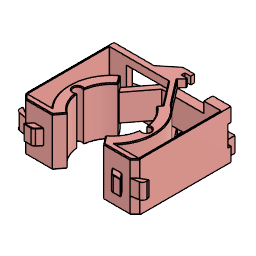
omega clamp - AS5311 (Autodesk Fusion 360 design; units mm, degrees)
Autodesk Fusion 360 part; units mm, degrees
sketch "Sketch1" plane through (0, 0, 0) normal (0, 0, 1) x (1, 0, 0)
  arc A0 (-9.9403, 13.1697) -> (-16.4122, 1.6998) centre (0, 0) ccw
  arc A1 (-16.4122, 1.6998) -> (-16.4122, -1.6998) centre (-17.8088, 0) ccw
  arc A2 (-16.4122, -1.6998) -> (-9.9403, -13.1697) centre (0, 0) ccw
  line L0 (0, 0) -> (-44, 0) construction
  arc A3 (-13.259, 17.5667) -> (-13.259, -17.5667) centre (0, 0) ccw
  line L1 (-9.9403, -13.1697) -> (-13.259, -17.5667)
  line L2 (-9.9403, 13.1697) -> (-13.259, 17.5667)
  line L3 (0, 0) -> (-9.9403, -13.1697) construction
  line L4 (0, 0) -> (-9.9403, 13.1697) construction
  point P0 (-20.0088, 0)
  point P1 (-16.0088, 0)
  point P2 (-22.0088, 0)
  dimension "d12" = 2.2
  dimension "d14" = 4
  dimension "d15" = 2
  dimension "d80" = 33
  dimension "d82" = 3.3997
  dimension "d83" = 105.91
  constraint coincident A0.centre A2.centre
  constraint horizontal L0
  constraint coincident A1.centre L0
  constraint midpoint A1 P0
  constraint coincident L0 P1
  constraint coincident L0 P2
  constraint coincident A3 P2
  constraint midpoint A3 P2
  constraint coincident A0.centre L1
  constraint parallel L2 L4
  constraint equal A0 A2
  measures "d12" radius of A1
  measures "d14" distance of P0 P1
  measures "d15" distance of P0 P2
  measures "d80" diameter of A0
  measures "d82" distance of A0.end A1.end
  measures "d83" angle of L3 L4
extrude "Extrude1" add sketch "Sketch1" along normal blind 25 makes body 1
mirror "Mirror1" about plane through (0, 0, 0) normal (1, 0, 0) of bodies 1 makes body 2
sketch "Sketch2" plane through (0, 0, 0) normal (0, 0, 1) x (1, 0, 0)
  arc A0 (-13.259, 17.5667) -> (-13.259, -17.5667) centre (0, 0) ccw
  arc A1 (-16.4122, -1.6998) -> (-9.9403, -13.1697) centre (0, 0) ccw
  arc A2 (-16.4122, 1.6998) -> (-16.4122, -1.6998) centre (-17.8088, 0) ccw
  arc A3 (-9.9403, 13.1697) -> (-16.4122, 1.6998) centre (0, 0) ccw
  arc A4 (16.4122, 1.6998) -> (9.9403, 13.1697) centre (0, 0) ccw
  arc A5 (16.4122, -1.6998) -> (16.4122, 1.6998) centre (17.8088, 0) ccw
  arc A6 (9.9403, -13.1697) -> (16.4122, -1.6998) centre (0, 0) ccw
  arc A7 (13.259, -17.5667) -> (13.259, 17.5667) centre (0, 0) ccw
  line L0 (-13.259, -17.5667) -> (-29.4985, -17.5667)
  line L1 (-29.4985, -17.5667) -> (-29.4985, -14.5667)
  line L2 (-29.4985, -14.5667) -> (-16.4985, -14.5667)
  line L3 (-29.4985, -14.5667) -> (-29.4985, 27.5667)
  line L4 (-28.8485, 27.5667) -> (-28.8485, -14.5667)
  line L5 (-29.4985, 27.5667) -> (1.7818, 27.5667)
  line L6 (-29.4985, 27.5667) -> (-29.4985, 30.5667)
  line L7 (-29.4985, 30.5667) -> (3.259, 30.5667)
  line L8 (3.259, 30.5667) -> (13.259, 17.5667)
  line L9 (1.7818, 27.5667) -> (11.3845, 15.0832)
  line L10 (-13.259, -17.5667) -> (-6.9615, -17.5667)
  line L11 (-26.9985, -17.5667) -> (-29.4985, -15.0667)
  line L12 (-6.9615, -17.5667) -> (36, -17.5667)
  line L13 (-9.9403, 13.1697) -> (-13.259, 17.5667)
  line L14 (-13.259, -17.5667) -> (-9.9403, -13.1697)
  line L15 (9.9403, -13.1697) -> (13.259, -17.5667)
  line L16 (13.259, 17.5667) -> (9.9403, 13.1697)
  dimension "d40" = 3
  dimension "d41" = 0.65
  dimension "d42" = 3
  dimension "d43" = 3
  dimension "d45" = 10
  dimension "d46" = 10
  dimension "d47" = 42.1333
  dimension "d48" = 13
  dimension "d49" = 45
  dimension "d50" = 0.5
  constraint horizontal L0
  constraint perpendicular L0 L1
  constraint coincident A0 L2.end
  constraint perpendicular L1 L2
  constraint perpendicular L2 L3
  constraint coincident L2 L4.end
  constraint perpendicular L2 L4
  constraint perpendicular L4 L5
  constraint coincident L4.start L5
  constraint perpendicular L5 L6
  constraint perpendicular L6 L7
  constraint coincident A7.end L8.end
  constraint parallel L8 L9
  constraint horizontal L10
  constraint coincident L0 L11.start
  constraint coincident L1 L11.end
  constraint parallel L10 L12
  constraint coincident L9.end L16
  constraint coincident A0.end L0.start
  measures "d40" distance of L0.end L1.end
  measures "d41" distance of L3 L4
  measures "d42" distance of L8 L9
  measures "d43" distance of L5 L7
  measures "d45" horizontal distance of L7.end A7.end
  measures "d46" vertical distance of A0.start L5.end
  measures "d47" distance of L1.end L3.end
  measures "d48" distance of L1.end L2.end
  measures "d49" angle of L0 L11
  measures "d50" distance of L1.end L11.end
extrude "Extrude2" add sketch "Sketch2" along normal up to surface (25 mm away) separate body contours A0 L0 L1 L2 L11 | L2 L3 L4 L5 | L5 L6 L7 L8 L9 L16 makes body 3
ref_plane "WorkPlane3" through (-8.1198, 6.5, 12.5) normal (0, 0, 1) x (1, 0, 0)
sketch "Sketch4" plane through (-6.4898, 5.5, 12.5) normal (0, 0, 1) x (1, 0, 0)
  line L0 (19.7488, 12.0667) -> (9.7488, 25.0667)
  line L1 (9.7488, 25.0667) -> (-23.0087, 25.0667)
  line L2 (-23.0087, 25.0667) -> (-23.0087, -20.5667)
  line L3 (-23.0087, -20.5667) -> (-20.5087, -23.0667)
  line L4 (-20.5087, -23.0667) -> (-6.7692, -23.0667)
  arc A0 (-10.0087, -20.0667) -> (-6.7692, -23.0667) centre (6.4898, -5.5) ccw
  line L5 (-20.5087, -23.0667) -> (-24.597, -22.3458)
  line L6 (-26.2193, -20.0289) -> (-26.0087, -18.8346)
  line L7 (-26.0087, -18.8346) -> (-23.0087, -20.5667)
  arc A1 (-26.2193, -20.0289) -> (-24.597, -22.3458) centre (-24.2497, -20.3762) ccw
  line L8 (17.8743, 9.5832) -> (19.7488, 12.0667)
  line L9 (-10.0087, -20.0667) -> (-22.3587, -20.0667)
  line L10 (-22.3587, -20.0667) -> (-22.3587, 22.0667)
  line L11 (-22.3587, 22.0667) -> (8.2716, 22.0667)
  line L12 (8.2716, 22.0667) -> (17.8743, 9.5832)
  line L13 (-16.2943, -23.0667) -> (-18.8116, -26.0667)
  line L14 (-18.8116, -26.0667) -> (-14.7443, -26.0667)
  arc A2 (-14.7443, -26.0667) -> (-13.2122, -25.3523) centre (-14.7443, -24.0667) ccw
  line L15 (-13.2122, -25.3523) -> (-11.2943, -23.0667)
  arc A3 (-18.5359, -25.7381) -> (-18.3827, -26.0667) centre (-18.3827, -25.8667) ccw
  dimension "d69" = 2
  dimension "d70" = 3
  dimension "d72" = 60
  dimension "d73" = 10
  dimension "d119" = 50
  dimension "d120" = 3
  dimension "d123" = 2
  dimension "d124" = 5
  dimension "d125" = 0.2
  constraint coincident L3.end L4.start
  constraint perpendicular L5 L6
  constraint coincident L2.end L3.start
  constraint tangent L5 A1
  constraint tangent L6 A1
  constraint coincident L4 L13.start
  constraint horizontal L14
  constraint tangent L14 A2
  constraint coincident L4 L15.end
  constraint parallel L13 L15
  constraint tangent A2 L15
  constraint tangent L13 A3
  constraint coincident L13 A3.start
  constraint coincident L14 A3.end
  constraint tangent L14 A3
  measures "d69" radius of A1
  measures "d70" horizontal distance of L6.end L2.end
  measures "d72" angle of L2 L7
  measures "d73" angle of L4 L5
  measures "d119" angle of L4 L13
  measures "d120" distance of L4 L13.end
  measures "d123" radius of A2
  measures "d124" distance of L13.start L15.end
  measures "d125" radius of A3
extrude "Extrude7" add sketch "Sketch4" along normal mid plane 8 contours L3 L5 L6 L7 A1 | L4 L13 L14 A2 L15 A3 bodies 3
mirror "Mirror2" about plane through (0, 0, 0) normal (1, 0, 0) of bodies 3 makes body 4
ref_plane "WorkPlane5" through (-13.1198, 30.5667, 12.5) normal (0, 1, 0) x (-1, 0, 0)
sketch "Sketch3" plane through (-13.1198, 30.5667, 12.5) normal (0, 1, 0) x (-1, 0, 0)
  line L0 (16.3787, -8.5) -> (-42.6183, -8.5)
  line L1 (16.3787, -6.9) -> (-42.6183, -6.9)
  line L2 (-42.6183, 6.9) -> (16.3787, 6.9)
  line L3 (16.3787, 8.5) -> (-43, 8.5)
  line L4 (-13.1198, -8.5) -> (-13.1198, -6.9) construction
  line L5 (-13.1198, -8.5) -> (-13.1198, -12.5) construction
  line L6 (6.8802, 12.5) -> (6.8802, -12.5)
  line L7 (-33.1198, -12.5) -> (-33.1198, 12.5)
  line L8 (-13.1198, -6.9) -> (-13.1198, 6.9) construction
  line L9 (-13.1198, 6.9) -> (-13.1198, 8.5) construction
  line L10 (-13.1198, 12.5) -> (-13.1198, 8.5) construction
  line L11 (-33.1198, -12.5) -> (6.8802, 12.5) construction
  line L12 (-42.6183, -12.5) -> (-42.6183, 12.5)
  line L13 (16.3787, -12.5) -> (16.3787, 12.5)
  line L14 (16.3787, -12.5) -> (-42.6183, -12.5)
  line L15 (-42.6183, 12.5) -> (16.3787, 12.5)
  point P0 (-13.1198, 0)
  dimension "d58" = 1.6
  dimension "d129" = 4
  dimension "d130" = 40
  constraint horizontal L2
  constraint vertical L4
  constraint vertical L5
  constraint coincident L2 L8.end
  constraint coincident L3 L9.end
  constraint vertical L6
  constraint vertical L7
  constraint coincident L0 L4.start
  constraint coincident L1 L4.end
  constraint equal L5 L10
  constraint equal L4 L9
  constraint vertical L8
  constraint vertical L9
  constraint vertical L10
  constraint midpoint L11 P0
  constraint coincident L8 P0
  constraint coincident L13.start L14.start
  constraint coincident L12.start L14.end
  constraint coincident L12.end L15.start
  constraint coincident L13.end L15.end
  constraint midpoint L5.end L14
  constraint horizontal L1
  constraint coincident L1.end L12
  constraint coincident L0.end L12
  constraint coincident L1.start L13
  constraint coincident L0.start L13
  constraint coincident L2.start L12
  constraint perpendicular L3 L12
  constraint midpoint L10.start L15
  constraint coincident L6.end L14
  constraint coincident L2.end L13
  constraint coincident L3.start L13
  constraint coincident L7.end L15
  constraint coincident L7.start L14
  constraint coincident L6.start L15
  measures "d58" distance of L0 L1
  measures "d129" distance of L4.start L5.end
  measures "d130" distance of L6 L7
extrude "Extrude5" cut sketch "Sketch3" against normal blind 20 contours L0 L6 L13 L14 | L0 L1 L6 L13 | L0 L6 L7 L14 | L0 L1 L6 L7 | L1 L2 L6 L13 | L2 L3 L6 L13 | L2 L3 L6 L7 | L3 L6 L13 L15 | L3 L6 L7 L15 bodies 4
extrude "Extrude6" cut sketch "Sketch3" against normal blind 25 contours L0 L1 L6 L7 | L1 L2 L6 L7 | L2 L3 L6 L7 bodies 3
combine "Combine1" operation add target body 1 tool bodies 2 3 4
sketch "Sketch5" plane through (0, 30.5667, 0) normal (0, 1, 0) x (-1, 0, 0)
  line L0 (-29.4985, 25) -> (-29.4985, 0)
  line L1 (-20, 0) -> (-20, 5.6)
  line L2 (-20, 5.6) -> (3.259, 5.6)
  line L3 (3.259, 5.6) -> (3.259, 19.4)
  line L4 (3.259, 19.4) -> (-20, 19.4)
  line L5 (3.259, 7.2) -> (-29.4985, 7.2)
  line L6 (3.259, 17.8) -> (-29.4985, 17.8)
  line L7 (3.259, 17.8) -> (-29.4985, 7.2) construction
  line L8 (-13.1198, 12.5) -> (3.259, 12.5) construction
  line L9 (-20, 25) -> (-29.4985, 25)
  line L10 (-29.4985, 0) -> (-20, 0)
  line L11 (-20, 19.4) -> (-20, 25)
  dimension "d84" = 10.6
  constraint coincident L3 L5.start
  constraint coincident L0 L5.end
  constraint perpendicular L0 L5
  constraint coincident L3 L6.start
  constraint coincident L0 L6.end
  constraint perpendicular L0 L6
  constraint midpoint L7 L8.start
  constraint midpoint L3 L8.end
  constraint horizontal L8
  measures "d84" distance of L5 L6
extrude "Extrude8" add sketch "Sketch5" along normal blind 1.6 contours L0 L3 L4 L6 L9 L11 | L0 L1 L2 L3 L5 L10 bodies 1
sketch "Sketch6" plane through (0, 0, 0) normal (0, 0, 1) x (1, 0, 0)
  line L0 (2.4985, 33.4667) -> (24.4985, 33.4667)
  line L1 (24.4985, 33.4667) -> (24.4985, 35.2667)
  line L2 (24.4985, 35.2667) -> (2.4985, 35.2667)
  line L3 (2.4985, 35.2667) -> (2.4985, 33.4667)
  line L4 (-3.259, 32.1667) -> (29.4985, 32.1667)
  line L5 (26.4985, 32.8667) -> (-29.4985, 32.8667)
  line L6 (-29.4985, 32.8667) -> (-29.4985, 37.2667)
  line L7 (-29.4985, 37.2667) -> (26.4985, 37.2667)
  line L8 (26.4985, 37.2667) -> (26.4985, 32.8667)
  arc A0 (-9.9403, 13.1697) -> (-16.4122, 1.6998) centre (0, 0) ccw
  arc A1 (-16.4122, 1.6998) -> (-16.4122, -1.6998) centre (-17.8088, 0) ccw
  arc A2 (-16.4122, -1.6998) -> (-9.9403, -13.1697) centre (0, 0) ccw
  line L9 (-9.9403, -13.1697) -> (-13.259, -17.5667)
  line L10 (-13.259, -17.5667) -> (-26.9985, -17.5667)
  line L11 (-26.9985, -17.5667) -> (-29.4985, -15.0667)
  line L12 (-29.4985, -15.0667) -> (-29.4985, 30.5667)
  line L13 (-29.4985, 30.5667) -> (3.259, 30.5667)
  line L14 (3.259, 30.5667) -> (13.259, 17.5667)
  arc A3 (16.4985, -14.5667) -> (13.259, 17.5667) centre (0, 0) ccw
  line L15 (16.4985, -14.5667) -> (28.8485, -14.5667)
  line L16 (28.8485, -14.5667) -> (28.8485, 27.5667)
  line L17 (28.8485, 27.5667) -> (20, 27.5667)
  line L18 (20, 27.5667) -> (20, 32.1667)
  line L19 (20, 32.1667) -> (29.4985, 32.1667)
  line L20 (29.4985, 32.1667) -> (29.4985, -15.0667)
  line L21 (29.4985, -15.0667) -> (26.9985, -17.5667)
  line L22 (26.9985, -17.5667) -> (13.259, -17.5667)
  line L23 (13.259, -17.5667) -> (9.9403, -13.1697)
  arc A4 (9.9403, -13.1697) -> (16.4122, -1.6998) centre (0, 0) ccw
  arc A5 (16.4122, -1.6998) -> (16.4122, 1.6998) centre (17.8088, 0) ccw
  arc A6 (16.4122, 1.6998) -> (9.9403, 13.1697) centre (0, 0) ccw
  line L24 (9.9403, 13.1697) -> (11.3845, 15.0832)
  line L25 (11.3845, 15.0832) -> (1.7818, 27.5667)
  line L26 (1.7818, 27.5667) -> (-28.8485, 27.5667)
  line L27 (-28.8485, 27.5667) -> (-28.8485, -14.5667)
  line L28 (-28.8485, -14.5667) -> (-16.4985, -14.5667)
  arc A7 (-13.259, 17.5667) -> (-16.4985, -14.5667) centre (0, 0) ccw
  line L29 (-13.259, 17.5667) -> (-9.9403, 13.1697)
  line L30 (-29.4985, 30.5667) -> (-29.4985, 32.8667)
  line L31 (3.259, 30.5667) -> (3.259, 32.8667)
  line L32 (-20, 30.5667) -> (-20, 27.5667)
  line L33 (-20, 30.5667) -> (-20, 32.8667)
  line L34 (-29.4985, 32.8667) -> (-9.4985, 37.2667)
  line L35 (18.4985, 35.2667) -> (18.4985, 33.4667)
  line L36 (8.4985, 33.4667) -> (8.4985, 35.2667)
  line L37 (8.4985, 33.4667) -> (18.4985, 35.2667) construction
  line L38 (13.4985, 34.3667) -> (13.4985, 35.2667) construction
  line L39 (5.4985, 32.8667) -> (5.4985, 33.4667)
  line L40 (5.4985, 35.2667) -> (5.4985, 37.2667)
  line L41 (-0.5015, 37.2667) -> (-8.741, 30.5667)
  line L42 (5.4985, 32.8667) -> (3.259, 30.5667)
  point P0 (3.259, 30.5667)
  dimension "d87" = 22
  dimension "d88" = 1.8
  dimension "d89" = 3.1
  dimension "d90" = 5
  dimension "d91" = 0.6
  dimension "d92" = 2
  dimension "d93" = 2
  dimension "d96" = 20
  dimension "d101" = 10
  dimension "d104" = 3
  dimension "d106" = 12
  dimension "d107" = 3
  constraint horizontal L0
  constraint vertical L1
  constraint horizontal L2
  constraint vertical L3
  constraint horizontal L5
  constraint vertical L6
  constraint horizontal L7
  constraint vertical L8
  constraint coincident L12.end L13.start
  constraint vertical L30
  constraint coincident P0 L13.end
  constraint coincident L5 L31.end
  constraint perpendicular L5 L31
  constraint coincident L5 L33.end
  constraint perpendicular L5 L33
  constraint coincident L32.start L33.start
  constraint coincident L7 L34.end
  constraint coincident L2 L35.start
  constraint coincident L0 L35.end
  constraint perpendicular L0 L35
  constraint coincident L0 L36.start
  constraint coincident L2 L36.end
  constraint perpendicular L2 L36
  constraint midpoint L37 L38.start
  constraint midpoint L2 L38.end
  constraint vertical L38
  constraint coincident L5 L39.start
  constraint coincident L0 L39.end
  constraint perpendicular L0 L39
  constraint coincident L2 L40.start
  constraint coincident L7 L40.end
  constraint perpendicular L7 L40
  constraint collinear L39 L40
  constraint coincident L7 L41.start
  constraint coincident L13 L41.end
  measures "d87" distance of L1.end L2.end
  measures "d88" distance of L0.start L2.end
  measures "d89" distance of L2 L4
  measures "d90" distance of L1 L4.end
  measures "d91" distance of L0 L5
  measures "d92" distance of L1 L8
  measures "d93" distance of L2 L7
  measures "d96" distance of L6.end L34.end
  measures "d101" distance of L35 L36
  measures "d104" distance of L3 L40
  measures "d106" distance of P0 L41.end
  measures "d107" horizontal distance of L2.end L41.start
extrude "Extrude9" add sketch "Sketch6" along normal blind 8 contours L0 L2 L3 L5 L7 L39 L40 L41 | L0 L1 L2 L5 L7 L8 L39 L40 | L5 L7 L34 L41 | L5 L13 L30 L33 bodies 1
extrude "Extrude10" add sketch "Sketch6" along normal up to surface (4 mm away) contours L5 L13 L31 L41 | L5 L13 L33 L41 bodies 1
ref_plane "WorkPlane4" through (13.1198, 31.3667, 12.5) normal (0, 0, 1) x (1, 0, 0)
extrude "Extrude11" add sketch "Sketch6" along normal up to surface (6 mm away) contours L0 L2 L3 L36 | L0 L1 L2 L35 bodies 1
extrude "Extrude12" add sketch "Sketch6" along normal up to surface (5 mm away) contours L0 L2 L35 L36 bodies 1
extrude "Extrude13" add sketch "Sketch6" along normal up to surface (4 mm away) from surface at 21 contours L0 L2 L3 L5 L7 L39 L40 L41 | L4 L5 L31 L42 | L5 L13 L31 L41 | L4 L31 L42 bodies 1
sketch "Sketch7" plane through (0, 30.5667, 0) normal (0, 1, 0) x (-1, 0, 0)
  line L0 (8.741, 25) -> (8.741, 21)
  line L1 (8.741, 21) -> (20, 21)
  line L2 (20, 21) -> (20, 8)
  line L3 (20, 8) -> (29.4985, 8)
  line L4 (29.4985, 8) -> (29.4985, 25)
  line L5 (29.4985, 25) -> (8.741, 25)
  line L6 (22.7493, 8) -> (24.7493, 12)
  line L7 (24.7493, 12) -> (26.7493, 8)
  line L8 (24.7493, 12) -> (24.7493, 8) construction
  dimension "d111" = 4
  dimension "d112" = 4
  constraint coincident L3 L6.start
  constraint coincident L3 L7.end
  constraint equal L6 L7
  constraint midpoint L3 L8.end
  constraint vertical L8
  measures "d111" distance of L6.end L8.end
  measures "d112" distance of L6.start L7.end
extrude "Extrude14" cut sketch "Sketch7" against normal blind 4 contours L3 L6 L7 bodies 1
chamfer "Chamfer7" distance 0.4 angle 45 40 edges at (-28.2485, -16.3167, 0) (-20.1287, -17.5667, 0) (-11.5996, -15.3682, 0) (-14.3702, -8.1085, 0) (-20.0088, 0, 0) (-14.3702, 8.1085, 0) (-11.5996, 15.3682, 0) (-21.8978, 2.2076, 0) (-22.6735, -14.5667, 0) (11.5996, -15.3682, 0) (20.1287, -17.5667, 0) (22.6735, -14.5667, 0) (28.2485, -16.3167, 0) (21.8978, 2.2076, 0) (14.3702, -8.1085, 0) (20.0088, 0, 0) (14.3702, 8.1085, 0) (10.6624, 14.1264, 0) (6.5831, 21.3249, 0) (8.259, 24.0667, 0) (8.259, 24.0667, 25) (6.5831, 21.3249, 25) (21.8978, 2.2076, 25) (10.6624, 14.1264, 25) (14.3702, 8.1085, 25) (20.0088, 0, 25) (14.3702, -8.1085, 25) (11.5996, -15.3682, 25) (20.1287, -17.5667, 25) (22.6735, -14.5667, 25) (28.2485, -16.3167, 25) (-20.1287, -17.5667, 25) (-28.2485, -16.3167, 25) (-22.6735, -14.5667, 25) (-21.8978, 2.2076, 25) (-14.3702, -8.1085, 25) (-11.5996, -15.3682, 25) (-20.0088, 0, 25) (-14.3702, 8.1085, 25) (-11.5996, 15.3682, 25) on bodies 1
chamfer "Chamfer6" distance 0.2 angle 45 24 edges at (-30.9985, -14.2006, 16.5) (-30.9985, -14.2006, 8.5) (-23.905, -18.9024, 8.5) (-25.0538, -20.4512, 8.5) (-23.0533, -20.5667, 8.5) (-20.3888, -20.3793, 8.5) (-18.7431, -18.7095, 8.5) (-23.905, -18.9024, 16.5) (-25.0538, -20.4512, 16.5) (-23.0533, -20.5667, 16.5) (-20.3888, -20.3793, 16.5) (-18.7431, -18.7095, 16.5) (18.7431, -18.7095, 16.5) (20.3888, -20.3793, 16.5) (23.0533, -20.5667, 16.5) (25.0538, -20.4512, 16.5) (23.905, -18.9024, 16.5) (18.7431, -18.7095, 8.5) (20.3888, -20.3793, 8.5) (23.0533, -20.5667, 8.5) (25.0538, -20.4512, 8.5) (23.905, -18.9024, 8.5) (30.9985, -14.2006, 16.5) (30.9985, -14.2006, 8.5) on bodies 1
equation "rubber_width = 29.5 mm"
equation "shaft_diameter = 33 mm"
equation "chord_angle = ( ( rubber_width + slop ) / ( shaft_diameter * PI ) * 2 * PI ) * 1 rad"
equation "d80 = shaft_diameter"
equation "slop = 1 mm"
equation "d83 = chord_angle"
named bodies: "omega clamp"
